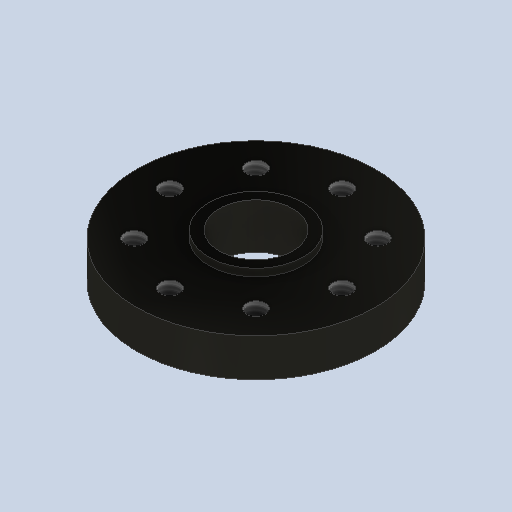
# Autodesk Inventor part: Servo_horn_Bottom
Saved by Autodesk Inventor 2023 (Build 270158000, 158)
## iProperties
Created: 2022-09-18
Part Number: Servo_horn_Bottom
Material: 일반
Document SubType Name: Modeling
Designer: 박동준
Density: 1 g/cm^3
Appearance: 기본값
품번: 7
Author: 박동준
Autodesk Inventor part; units mm, degrees
ref_plane "YZ Plane" through (0, 0, 0) normal (1, 0, 0) x (0, 1, 0)
ref_plane "XZ Plane" through (0, 0, 0) normal (0, 1, 0) x (-1, 0, 0)
ref_plane "XY Plane" through (0, 0, 0) normal (0, 0, 1) x (1, 0, 0)
sketch "스케치1" plane through (0, 0, 0) normal (0, 0, 1) x (1, 0, 0)
  line L0 (0, 8.1862) -> (0, -8.1862)
  line L1 (3, 1.85) -> (3.85, 1.85)
  line L2 (3.85, 1.85) -> (3.85, 1.25)
  line L3 (3.85, 1.25) -> (9.75, 1.25)
  line L4 (9.75, 1.25) -> (9.75, -1.85)
  line L5 (9.75, -1.85) -> (3, -1.85)
  line L6 (3, -1.85) -> (3, 1.85)
  point P0 (0, 0)
  point P1 (0, 0)
  point P2 (6.8, 1.25)
  point P3 (3, 0)
  dimension "d0" = 6
  dimension "d1" = 7.7
  dimension "d2" = 19.5
  dimension "d3" = 0.6
  dimension "d4" = 3.1
  constraints: 14 end point, 5 perpendicular, 3 midpoint, 1 coincident, 1 horizontal, 1 horizontal alignment, 1 vertical
  measures "d0" diameter of L6 L0
  measures "d1" diameter of L2 L0
  measures "d2" diameter of L4 L0
  measures "d3" distance from line of point (6.8, 1.25) L1
  measures "d4" distance between parallel lines of L5 L3
revolve "회전1" add sketch "스케치1" angle 360 about axis through (0, 8.1862, 0) along (0, -1, 0)
sketch "스케치2" plane through (0, 1.25, 0) normal (0, 1, 0) x (1, 0, 0)
  circle A0 centre (0, 0) radius 3.85 projected
  circle A1 centre (0, 0) radius 9.75 projected
  circle A2 centre (0, 0) radius 3 projected
  point P0 (0, 0)
  point P1 (7.025, 0)
  point P2 (4.9674, 4.9674)
  point P3 (0, 7.025)
  point P4 (-4.9674, 4.9674)
  point P5 (-7.025, 0)
  point P6 (-4.9674, -4.9674)
  point P7 (0, -7.025)
  point P8 (4.9674, -4.9674)
  dimension "d6" = 7.025
  dimension "d9" = 360
  constraints: 9 other
  measures "d6" distance of point (7.025, 0) point (0, 0)
hole "구멍1" at (7.025, 1.25, 0) at (4.9674, 1.25, -4.9674) at (0, 1.25, -7.025) at (-4.9674, 1.25, -4.9674) at (-7.025, 1.25, 0) at (-4.9674, 1.25, 4.9674) at (0, 1.25, 7.025) at (4.9674, 1.25, 4.9674) direction (0, -1, 0) diameter 1.567 end through all thread size "M2x0.4" class "6H" standard "ISO Metric profile"
